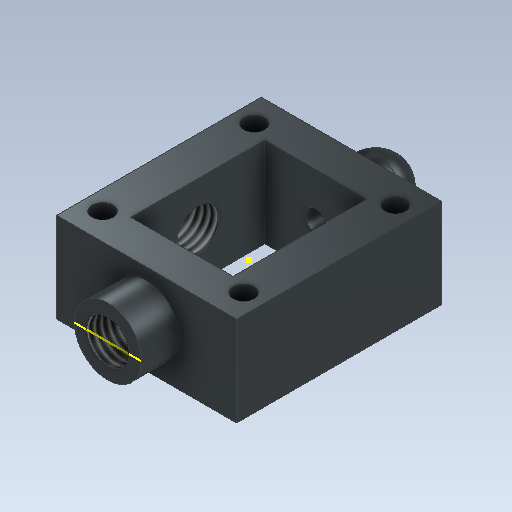
# Autodesk Inventor part: Part4
Saved by Autodesk Inventor 2020 (Build 240168000, 168)
## iProperties
Created: 2021-10-13
Part Number: Part4
Material: Iron, Cast
Document SubType Name: Modeling
Designer: simon.erikssonwestl
Density: 7.15 g/cm^3
Appearance: Iron Gray
Author: simon.erikssonwestl
Autodesk Inventor part; units mm, degrees
ref_plane "YZ Plane" through (0, 0, 0) normal (1, 0, 0) x (0, 1, 0)
ref_plane "XZ Plane" through (0, 0, 0) normal (0, 1, 0) x (-1, 0, 0)
ref_plane "XY Plane" through (0, 0, 0) normal (0, 0, 1) x (1, 0, 0)
sketch "Sketch1" plane through (0, 0, 0) normal (0, 1, 0) x (-1, 0, 0)
  line L0 (12.75, -14.5) -> (-12.75, -14.5)
  line L1 (-12.75, -14.5) -> (-12.75, 14.5)
  line L2 (-12.75, 14.5) -> (12.75, 14.5)
  line L3 (12.75, 14.5) -> (12.75, -14.5)
  line L4 (12.75, -14.5) -> (-12.75, 14.5) construction
  line L5 (-12.75, -14.5) -> (12.75, 14.5) construction
  point P0 (0, 0)
  dimension "d0" = 25.5
  dimension "d1" = 29
  constraints: 12 end point, 2 midpoint, 2 parallel, 1 horizontal, 1 perpendicular
  measures "d0" distance of L1.end L2.end
  measures "d1" distance of L0.end L1.end
extrude "Extrusion1" add sketch "Sketch1" along normal mid plane 12.75
sketch "Sketch2" plane through (0, 6.375, 0) normal (0, 1, 0) x (1, 0, 0)
  line L0 (-7.25, 9.5) -> (7.25, 9.5)
  line L1 (7.25, 9.5) -> (7.25, -9.5)
  line L2 (7.25, -9.5) -> (-7.25, -9.5)
  line L3 (-7.25, -9.5) -> (-7.25, 9.5)
  line L4 (-7.25, 9.5) -> (7.25, -9.5) construction
  line L5 (7.25, 9.5) -> (-7.25, -9.5) construction
  point P0 (0, 0)
  dimension "d4" = 14.5
  dimension "d5" = 19
  constraints: 12 end point, 2 midpoint, 2 parallel, 1 horizontal, 1 perpendicular
  measures "d4" distance of L1.end L2.end
  measures "d5" distance of L0.end L1.end
extrude "Extrusion2" cut sketch "Sketch2" against normal blind 12.75
sketch "Sketch3" plane through (0, 6.375, 0) normal (0, 1, 0) x (1, 0, 0)
  circle A0 centre (10, 10.75) radius 1.5
  line L0 (12.75, 14.5) -> (-12.75, 14.5) projected
  line L1 (12.75, -14.5) -> (12.75, 14.5) projected
  circle A1 centre (-10, 10.75) radius 1.5
  circle A2 centre (10, -10.75) radius 1.5
  circle A3 centre (-10, -10.75) radius 1.5
  point P0 (0, 0)
  dimension "d8" = 3
  dimension "d9" = 3.75
  dimension "d10" = 2.75
  dimension "d13" = 20
  dimension "d16" = 21.5
  constraints: 4 centre point, 1 horizontal, 1 vertical, 6 other
  measures "d8" diameter of A0
  measures "d9" distance from line of L0 A0.centre
  measures "d10" distance from line of L1 A0.centre
  measures "d13" distance of A0.centre A1.centre
  measures "d16" distance of A0.centre A2.centre
sketch "Sketch4" plane through (-12.75, 6.375, 14.5) normal (0, 0, 1) x (1, 0, 0)
  circle A0 centre (12.75, -6.375) radius 4.75
  dimension "d19" = 9.5
  constraints: 1 centre point, 1 coincident
  measures "d19" diameter of A0
extrude "Extrusion3" add sketch "Sketch4" along normal blind 5.5
extrude "Extrusion6" cut sketch "Sketch3" against normal through all
sketch "Sketch7" plane through (12.75, 6.375, -14.5) normal (0, 0, -1) x (-1, 0, 0)
  circle A0 centre (12.75, -6.375) radius 1.2632
  circle A1 centre (12.75, -6.375) radius 4
  point P0 (12.75, -6.375)
  dimension "d32" = 8
  constraints: 2 centre point, 1 coincident
  measures "d32" diameter of A1
extrude "Extrusion7" add sketch "Sketch7" along normal blind 7.5 contours A0 | A1
sketch "Sketch8" plane through (-12.75, -6.375, 14.5) normal (-1, 0, 0) x (0, 0, 1)
  circle A0 centre (-14.5, 6.375) radius 3
  dimension "d35" = 6
  constraints: 1 centre point, 1 coincident
  measures "d35" diameter of A0
hole "Hole1" at (-12.75, 0, 0) direction (1, 0, 0) diameter 6 depth 8 tip angle 118
thread "Thread2" size "M6x1" class "6H" standard "ANSI Metric M Profile" full length
fillet "Fillet1" [suppressed]
sketch "Sketch10" plane through (0, 0, 20) normal (0, 0, 1) x (1, 0, 0)
  circle A0 centre (0, 0) radius 1.5 projected
  point P0 (0, 0)
  constraints: 1 coincident
hole "Hole2" at (0, 0, 20) direction (0, 0, -1) diameter 6 depth 6 tip angle 118
sketch "Sketch11" plane through (7.25, 6.375, 9.5) normal (0, 0, -1) x (-1, 0, 0)
  circle A0 centre (7.25, -6.375) radius 1.5 projected
  constraints: 2 coincident
hole "Hole3" at (0, 0, 9.5) direction (0, 0, 1) diameter 3 end through all
thread "Thread3" size "M6x1" class "6H" standard "ANSI Metric M Profile" full length
fillet "Fillet2" radius 4 1 edges at (4, 0, -22)
sketch "Sketch12" plane through (-7.25, 6.375, -9.5) normal (0, 0, 1) x (1, 0, 0)
  point P0 (7.25, -6.375)
  point P1 (7.25, -6.375)
  constraints: 1 coincident
sketch "Sketch13" plane through (0, 0, 0) normal (0, 1, 0) x (-1, 0, 0)
  line L0 (-4, -18) -> (4, -18) projected
  line L1 (4.75, 20) -> (-4.75, 20) projected
  point P0 (0, 0)
  point P1 (0, -18)
  dimension "d67" = 38
  measures "d67" distance from line of L1 point (0, -18)
hole "Hole4" at (0, 0, -9.5) direction (0, 0, -1) diameter 3 depth 8.5 tip angle 118
body "Solid1"
